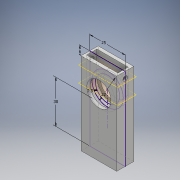
# Autodesk Inventor part: connecting_rod_crankschaft_side
Saved by Autodesk Inventor 2018 (Build 220112000, 112)
## iProperties
Created: 2026-05-03
Part Number: connecting_rod_crankschaft_side
Material: Generic
Document SubType Name: Modeling
Designer: neo
Density: 1 g/cm^3
Appearance: Default
Author: neo
Autodesk Inventor part; units mm, degrees
ref_plane "YZ Plane" through (0, 0, 0) normal (1, 0, 0) x (0, 1, 0)
ref_plane "XZ Plane" through (0, 0, 0) normal (0, 1, 0) x (-1, 0, 0)
ref_plane "XY Plane" through (0, 0, 0) normal (0, 0, 1) x (1, 0, 0)
sketch "Sketch1" plane through (0, 0, 0) normal (0, 1, 0) x (-1, 0, 0)
  circle A0 centre (0, 0) radius 11
  line L0 (0, 0) -> (0, -24.9996)
  line L1 (12.5, 17) -> (-12.5, 17)
  line L2 (-12.5, 17) -> (-12.5, -41)
  line L3 (-12.5, -41) -> (12.5, -41)
  line L4 (12.5, -41) -> (12.5, 17)
  circle A1 centre (0, 0) radius 8.5
  line L5 (0, 11) -> (9.8279, 11) construction
  line L6 (0, -11) -> (10.2574, -11) construction
  dimension "d0" = 22
  dimension "d1" = 2.5
  dimension "d2" = 25
  dimension "d3" = 6
  dimension "d4" = 30
  constraints: 14 end point, 3 horizontal, 2 centre point, 2 coincident, 2 parallel, 2 point on circle, 2 tangent, 1 perpendicular, 1 point on line, 1 vertical, 1 other
  measures "d0" diameter of A0
  measures "d1" radial gap between concentric circles of A0 A1
  measures "d2" distance of L1.start L1.end
  measures "d3" distance between parallel lines of L1 L5
  measures "d4" distance between parallel lines of L3 L6
extrude "Extrusion1" add sketch "Sketch1" along normal mid plane 12 contours A0 | L4 L3 L2 L1
extrude "Extrusion2" cut sketch "Sketch1" along normal mid plane 7.2 contours A0
sketch "Sketch2" plane through (-12.5, 6, 17) normal (0, 0, 1) x (1, 0, 0)
  line L0 (1.5, -9.6) -> (1.5, -2.4) projected
  line L1 (23.5, -9.6) -> (23.5, -2.4) projected
  line L2 (23.5, -2.4) -> (1.5, -2.4) projected
  line L3 (1.5, -9.6) -> (23.5, -9.6) projected
  point P0 (12.5, -6)
ref_plane "Work Plane1" through (0, 0, 0) normal (0, 0, 1) x (1, 0, 0)
extrude "Extrusion3" cut sketch "Sketch2" against normal up to surface (17 mm away)
ref_plane "Work Plane2" through (0, 0, 11) normal (0, 0, 1) x (1, 0, 0)
sketch "Sketch3" plane through (12.5, -6, -41) normal (1, 0, 0) x (0, 0, -1)
  line L0 (-52, -2.4) -> (-52, 14.4) construction
  circle A0 centre (-53.6, 6) radius 1.6
  point P0 (-41, 6)
  dimension "d11" = 3.2
  constraints: 1 centre point, 1 tangent
  measures "d11" diameter of A0
extrude "Extrusion4" cut sketch "Sketch3" against normal through all
body "Solid1"
